Autodesk Fusion 360 part; units mm, degrees
note: some values were not read from the file. Set by a fixed rule: which sketch regions a step uses.
(part 2 of 2)
sketch "Lead ins" plane through (0, 0, 0) normal (0, 0, 1) x (1, 0, 0)
  line L0 (76.8702, 33.6176) -> (72.7083, 33.6176) construction
  line L1 (72.7083, 33.6176) -> (70, 33.6176)
  line L2 (-72.7083, 33.6176) -> (-76.8702, 33.6176) construction
  line L3 (-72.7083, 33.6176) -> (-70, 33.6176)
  line L4 (-70, 33.6176) -> (-70, 33.3926) construction
  line L5 (70, 33.6176) -> (70, 33.3926) construction
  line L6 (-72.7083, 8.1676) -> (-76.8702, 8.1676) construction
  arc A0 (-72.7083, 8.1676) -> (-68.9368, 10.4435) centre (-70, 7.9426) ccw construction
  arc A1 (-68.9368, 10.4435) -> (-72.7083, 8.1676) centre (-70, 7.9426) ccw construction
  arc A2 (-71.4041, 10.2693) -> (-72.7083, 8.1676) centre (-70, 7.9426) ccw
  line L7 (-72.7083, 8.1676) -> (-70, 8.1676)
  line L8 (-70, 7.9426) -> (-70, 8.1676) construction
  line L9 (76.8702, 8.1676) -> (72.7083, 8.1676) construction
  arc A3 (68.9368, 10.4435) -> (72.7083, 8.1676) centre (70, 7.9426) ccw construction
  line L10 (72.7083, 8.1676) -> (70, 8.1676)
  line L11 (70, 8.1676) -> (70, 7.9426) construction
  arc A4 (72.7083, 8.1676) -> (68.9368, 10.4435) centre (70, 7.9426) ccw construction
  arc A5 (72.7083, 8.1676) -> (71.4041, 10.2693) centre (70, 7.9426) ccw
  point P0 (-70, 33.3926)
  point P1 (70, 33.3926)
  point P2 (-70, 7.9426)
  point P3 (71.4041, 10.2693)
  constraint parallel L0 L1
  constraint coincident L2.start L3.start
  constraint parallel L2 L3
  constraint coincident P0 L4.end
  constraint perpendicular L3 L4
  constraint coincident P1 L5.end
  constraint perpendicular L1 L5
  constraint coincident L0.end L1.start
  constraint coincident L6.start A0.start
  constraint coincident A0.end A1.start
  constraint coincident P2 A0.centre
  constraint midpoint A1 A2.start
  constraint parallel L6 L7
  constraint perpendicular L7 L8
  constraint coincident L9.end A3.end
  constraint parallel L9 L10
  constraint coincident A3.centre L11.end
  constraint perpendicular L10 L11
  constraint coincident A3.start A4.end
  constraint midpoint A4 P3
  constraint coincident P3 A5.end
sketch "Cuts" plane through (0, 0, 0) normal (0, 0, 1) x (1, 0, 0)
  arc A0 (-60.4613, 48.9428) -> (-61.177, 48.6145) centre (-53.134, 32.0265) ccw
  line L0 (-61.177, 48.6145) -> (-61.2612, 48.783)
  arc A1 (-61.2612, 48.783) -> (-64.4705, 49.6307) centre (-63.2391, 47.794) ccw
  line L1 (-64.4705, 49.6307) -> (-66.6685, 48.1572)
  arc A2 (-66.6685, 48.1572) -> (-66.9278, 45.5047) centre (-65.7079, 46.7244) ccw
  line L2 (-66.9278, 45.5047) -> (-66.4745, 45.0513)
  line L3 (-66.4745, 45.0513) -> (-65.6771, 45.5859)
  line L4 (-65.6771, 45.5859) -> (-65.6567, 45.5555)
  arc A3 (-65.6567, 45.5555) -> (-70.2084, 38.9774) centre (-53.134, 32.0265) ccw
  arc A4 (-70.2084, 38.9774) -> (-68.9368, 35.8935) centre (-68.0067, 38.0811) ccw
  arc A5 (-72.7083, 33.6176) -> (-68.9368, 35.8935) centre (-70, 33.3926) ccw
  line L5 (-72.7083, 33.6176) -> (-76.8702, 33.6176)
  arc A6 (-76.8702, 33.6176) -> (-78.0824, 32.2161) centre (-76.8702, 32.3926) ccw
  arc A7 (-78.0824, 32.2161) -> (-70, 25.225) centre (-70, 33.3926) ccw
  line L6 (-70, 25.225) -> (-53.8183, 25.225)
  line L7 (-53.8183, 25.225) -> (-52.078, 25.5991)
  arc A8 (-52.078, 25.5991) -> (-51.2745, 26.1842) centre (-52.3354, 26.7967) ccw
  line L8 (-51.2745, 26.1842) -> (-50.3319, 27.817)
  arc A9 (-50.3319, 27.817) -> (-47.5143, 26.9115) centre (-46.5, 34.9039) ccw
  line L9 (-47.5143, 26.9115) -> (-45.4857, 26.9115)
  arc A10 (-45.4857, 26.9115) -> (-41.0636, 28.9581) centre (-46.5, 34.9039) ccw
  arc A11 (-41.0636, 28.9581) -> (-40.8293, 30.4746) centre (-41.8902, 29.8621) ccw
  line L10 (-40.8293, 30.4746) -> (-43.0033, 34.24)
  line L11 (-43.0033, 34.24) -> (-44.1175, 33.5967)
  arc A12 (-45.5402, 32.3615) -> (-44.1175, 33.5967) centre (-46.5, 34.9039) ccw
  line L12 (-45.5402, 32.3615) -> (-47.4598, 32.3615)
  arc A13 (-48.8317, 33.5081) -> (-47.4598, 32.3615) centre (-46.5, 34.9039) ccw
  arc A14 (-48.0318, 36.5907) -> (-48.8317, 33.5081) centre (-46.9147, 34.6557) ccw
  line L13 (-48.0318, 36.5907) -> (-43.7627, 39.0554)
  line L14 (-43.7627, 39.0554) -> (-39.2352, 31.2135)
  arc A15 (-39.2352, 31.2135) -> (-33.999, 28.6496) centre (-34.7102, 33.826) ccw
  arc A16 (-2.725, 30.9595) -> (-33.999, 28.6496) centre (0, -218.8006) ccw
  line L15 (-2.725, 30.9595) -> (-2.725, 31.7494)
  arc A17 (-1, 33.4744) -> (-2.725, 31.7494) centre (-1, 31.7494) ccw
  line L16 (-1, 33.4744) -> (1, 33.4744)
  arc A18 (2.725, 31.7494) -> (1, 33.4744) centre (1, 31.7494) ccw
  line L17 (2.725, 31.7494) -> (2.725, 30.9595)
  arc A19 (33.999, 28.6496) -> (2.725, 30.9595) centre (0, -218.8006) ccw
  arc A20 (33.999, 28.6496) -> (39.2352, 31.2135) centre (34.7102, 33.826) ccw
  line L18 (39.2352, 31.2135) -> (43.7627, 39.0554)
  line L19 (43.7627, 39.0554) -> (48.0318, 36.5907)
  arc A21 (48.8317, 33.5081) -> (48.0318, 36.5907) centre (46.9147, 34.6557) ccw
  arc A22 (47.4598, 32.3615) -> (48.8317, 33.5081) centre (46.5, 34.9039) ccw
  line L20 (47.4598, 32.3615) -> (45.5402, 32.3615)
  arc A23 (44.1175, 33.5967) -> (45.5402, 32.3615) centre (46.5, 34.9039) ccw
  line L21 (44.1175, 33.5967) -> (43.0033, 34.24)
  line L22 (43.0033, 34.24) -> (40.8293, 30.4746)
  arc A24 (40.8293, 30.4746) -> (41.0636, 28.9581) centre (41.8902, 29.8621) ccw
  arc A25 (41.0636, 28.9581) -> (45.4857, 26.9115) centre (46.5, 34.9039) ccw
  line L23 (45.4857, 26.9115) -> (47.5143, 26.9115)
  arc A26 (47.5143, 26.9115) -> (50.3319, 27.817) centre (46.5, 34.9039) ccw
  line L24 (50.3319, 27.817) -> (51.2745, 26.1842)
  arc A27 (51.2745, 26.1842) -> (52.078, 25.5991) centre (52.3354, 26.7967) ccw
  line L25 (52.078, 25.5991) -> (53.8183, 25.225)
  line L26 (53.8183, 25.225) -> (70, 25.225)
  arc A28 (70, 25.225) -> (78.0824, 32.2161) centre (70, 33.3926) ccw
  arc A29 (78.0824, 32.2161) -> (76.8702, 33.6176) centre (76.8702, 32.3926) ccw
  line L27 (76.8702, 33.6176) -> (72.7083, 33.6176)
  arc A30 (68.9368, 35.8935) -> (72.7083, 33.6176) centre (70, 33.3926) ccw
  arc A31 (68.9368, 35.8935) -> (70.2084, 38.9774) centre (68.0067, 38.0811) ccw
  arc A32 (70.2084, 38.9774) -> (65.6567, 45.5555) centre (53.134, 32.0265) ccw
  line L28 (65.6567, 45.5555) -> (65.6771, 45.5859)
  line L29 (65.6771, 45.5859) -> (66.4745, 45.0513)
  line L30 (66.4745, 45.0513) -> (66.9278, 45.5047)
  arc A33 (66.9278, 45.5047) -> (66.6685, 48.1572) centre (65.7079, 46.7244) ccw
  line L31 (66.6685, 48.1572) -> (64.4705, 49.6307)
  arc A34 (64.4705, 49.6307) -> (61.2612, 48.783) centre (63.2391, 47.794) ccw
  line L32 (61.2612, 48.783) -> (61.177, 48.6145)
  arc A35 (61.177, 48.6145) -> (60.4613, 48.9428) centre (53.134, 32.0265) ccw
  arc A36 (60.4613, 48.9428) -> (59.7108, 49.1956) centre (58.5833, 44.6071) ccw
  arc A37 (59.7108, 49.1956) -> (2.725, 56.4095) centre (0, -193.8006) ccw
  line L33 (2.725, 56.4095) -> (2.725, 57.1994)
  arc A38 (2.725, 57.1994) -> (1, 58.9244) centre (1, 57.1994) ccw
  line L34 (1, 58.9244) -> (-1, 58.9244)
  arc A39 (-1, 58.9244) -> (-2.725, 57.1994) centre (-1, 57.1994) ccw
  line L35 (-2.725, 57.1994) -> (-2.725, 56.4095)
  arc A40 (-59.7108, 49.1956) -> (-60.4613, 48.9428) centre (-58.5833, 44.6071) ccw
  arc A41 (-2.725, 56.4095) -> (-59.7108, 49.1956) centre (0, -193.8006) ccw
  arc A42 (-39.2352, 5.7635) -> (-33.999, 3.1996) centre (-34.7102, 8.376) ccw
  line L36 (-43.7627, 13.6054) -> (-39.2352, 5.7635)
  line L37 (-48.0318, 11.1407) -> (-43.7627, 13.6054)
  arc A43 (-48.0318, 11.1407) -> (-48.8317, 8.0581) centre (-46.9147, 9.2057) ccw
  arc A44 (-48.8317, 8.0581) -> (-47.4598, 6.9115) centre (-46.5, 9.4539) ccw
  line L38 (-45.5402, 6.9115) -> (-47.4598, 6.9115)
  arc A45 (-45.5402, 6.9115) -> (-44.1175, 8.1467) centre (-46.5, 9.4539) ccw
  line L39 (-43.0033, 8.79) -> (-44.1175, 8.1467)
  line L40 (-40.8293, 5.0246) -> (-43.0033, 8.79)
  arc A46 (-41.0636, 3.5081) -> (-40.8293, 5.0246) centre (-41.8902, 4.4121) ccw
  arc A47 (-45.4857, 1.4615) -> (-41.0636, 3.5081) centre (-46.5, 9.4539) ccw
  line L41 (-47.5143, 1.4615) -> (-45.4857, 1.4615)
  arc A48 (-50.3319, 2.367) -> (-47.5143, 1.4615) centre (-46.5, 9.4539) ccw
  line L42 (-51.2745, 0.7342) -> (-50.3319, 2.367)
  arc A49 (-52.078, 0.1491) -> (-51.2745, 0.7342) centre (-52.3354, 1.3467) ccw
  line L43 (-53.8183, -0.225) -> (-52.078, 0.1491)
  line L44 (-70, -0.225) -> (-53.8183, -0.225)
  arc A50 (-78.0824, 6.7661) -> (-70, -0.225) centre (-70, 7.9426) ccw
  arc A51 (-76.8702, 8.1676) -> (-78.0824, 6.7661) centre (-76.8702, 6.9426) ccw
  line L45 (-72.7083, 8.1676) -> (-76.8702, 8.1676)
  arc A52 (-72.7083, 8.1676) -> (-68.9368, 10.4435) centre (-70, 7.9426) ccw
  arc A53 (-70.2084, 13.5274) -> (-68.9368, 10.4435) centre (-68.0067, 12.6311) ccw
  arc A54 (-65.6567, 20.1055) -> (-70.2084, 13.5274) centre (-53.134, 6.5765) ccw
  line L46 (-65.6771, 20.1359) -> (-65.6567, 20.1055)
  line L47 (-66.4745, 19.6013) -> (-65.6771, 20.1359)
  line L48 (-66.9278, 20.0547) -> (-66.4745, 19.6013)
  arc A55 (-66.6685, 22.7072) -> (-66.9278, 20.0547) centre (-65.7079, 21.2744) ccw
  line L49 (-64.4705, 24.1807) -> (-66.6685, 22.7072)
  arc A56 (-61.2612, 23.333) -> (-64.4705, 24.1807) centre (-63.2391, 22.344) ccw
  line L50 (-61.177, 23.1645) -> (-61.2612, 23.333)
  arc A57 (-60.4613, 23.4928) -> (-61.177, 23.1645) centre (-53.134, 6.5765) ccw
  arc A58 (-59.7108, 23.7456) -> (-60.4613, 23.4928) centre (-58.5833, 19.1571) ccw
  arc A59 (60.4613, 23.4928) -> (59.7108, 23.7456) centre (58.5833, 19.1571) ccw
  arc A60 (61.177, 23.1645) -> (60.4613, 23.4928) centre (53.134, 6.5765) ccw
  line L51 (61.2612, 23.333) -> (61.177, 23.1645)
  arc A61 (64.4705, 24.1807) -> (61.2612, 23.333) centre (63.2391, 22.344) ccw
  line L52 (66.6685, 22.7072) -> (64.4705, 24.1807)
  arc A62 (66.9278, 20.0547) -> (66.6685, 22.7072) centre (65.7079, 21.2744) ccw
  line L53 (66.4745, 19.6013) -> (66.9278, 20.0547)
  line L54 (65.6771, 20.1359) -> (66.4745, 19.6013)
  line L55 (65.6567, 20.1055) -> (65.6771, 20.1359)
  arc A63 (70.2084, 13.5274) -> (65.6567, 20.1055) centre (53.134, 6.5765) ccw
  arc A64 (68.9368, 10.4435) -> (70.2084, 13.5274) centre (68.0067, 12.6311) ccw
  arc A65 (68.9368, 10.4435) -> (72.7083, 8.1676) centre (70, 7.9426) ccw
  line L56 (76.8702, 8.1676) -> (72.7083, 8.1676)
  arc A66 (78.0824, 6.7661) -> (76.8702, 8.1676) centre (76.8702, 6.9426) ccw
  arc A67 (70, -0.225) -> (78.0824, 6.7661) centre (70, 7.9426) ccw
  line L57 (53.8183, -0.225) -> (70, -0.225)
  line L58 (52.078, 0.1491) -> (53.8183, -0.225)
  arc A68 (51.2745, 0.7342) -> (52.078, 0.1491) centre (52.3354, 1.3467) ccw
  line L59 (50.3319, 2.367) -> (51.2745, 0.7342)
  arc A69 (47.5143, 1.4615) -> (50.3319, 2.367) centre (46.5, 9.4539) ccw
  line L60 (45.4857, 1.4615) -> (47.5143, 1.4615)
  arc A70 (41.0636, 3.5081) -> (45.4857, 1.4615) centre (46.5, 9.4539) ccw
  arc A71 (40.8293, 5.0246) -> (41.0636, 3.5081) centre (41.8902, 4.4121) ccw
  line L61 (43.0033, 8.79) -> (40.8293, 5.0246)
  line L62 (44.1175, 8.1467) -> (43.0033, 8.79)
  arc A72 (44.1175, 8.1467) -> (45.5402, 6.9115) centre (46.5, 9.4539) ccw
  line L63 (47.4598, 6.9115) -> (45.5402, 6.9115)
  arc A73 (47.4598, 6.9115) -> (48.8317, 8.0581) centre (46.5, 9.4539) ccw
  arc A74 (48.8317, 8.0581) -> (48.0318, 11.1407) centre (46.9147, 9.2057) ccw
  line L64 (43.7627, 13.6054) -> (48.0318, 11.1407)
  line L65 (39.2352, 5.7635) -> (43.7627, 13.6054)
  arc A75 (33.999, 3.1996) -> (39.2352, 5.7635) centre (34.7102, 8.376) ccw
  arc A76 (33.999, 3.1996) -> (2.725, 5.5095) centre (0, -244.2506) ccw
  line L66 (2.725, 6.2994) -> (2.725, 5.5095)
  arc A77 (2.725, 6.2994) -> (1, 8.0244) centre (1, 6.2994) ccw
  line L67 (-1, 8.0244) -> (1, 8.0244)
  arc A78 (-1, 8.0244) -> (-2.725, 6.2994) centre (-1, 6.2994) ccw
  line L68 (-2.725, 5.5095) -> (-2.725, 6.2994)
  arc A79 (-2.725, 5.5095) -> (-33.999, 3.1996) centre (0, -244.2506) ccw
  arc A80 (-2.725, 30.9595) -> (-59.7108, 23.7456) centre (0, -219.2506) ccw construction
  arc A81 (59.7108, 23.7456) -> (2.725, 30.9595) centre (0, -219.2506) ccw construction
  arc A82 (-34.3171, 28.61) -> (-59.7108, 23.7456) centre (0, -219.2506) ccw
  arc A83 (59.7108, 23.7456) -> (34.3171, 28.61) centre (0, -219.2506) ccw
  line L69 (72.7083, 8.1676) -> (70, 8.1676)
  arc A84 (72.7083, 8.1676) -> (71.4041, 10.2693) centre (70, 7.9426) ccw
  line L70 (72.7083, 33.6176) -> (70, 33.6176)
  point P0 (-34.2057, 28.6254)
  point P1 (-34.3171, 28.61)
  point P2 (34.2057, 28.6254)
  point P3 (34.3171, 28.61)
  dimension "d667" = 0.1125
  dimension "d668" = 0.1125
  constraint coincident A80 P0
  constraint coincident A15 P0
  constraint coincident A80 P1
  constraint coincident A58.start A80.end
  constraint coincident P1 A82.start
  constraint concentric A80 A82
  constraint coincident A20 P2
  constraint coincident A81 P2
  constraint coincident A81 P3
  constraint coincident P3 A83.end
  constraint coincident A59.end A81.start
  constraint concentric A81 A83
  measures "d667" distance of P0 P1
  measures "d668" distance of P2 P3
sketch "Sketch58" plane through (0, 0, 3) normal (0, 0, 1) x (-1, 0, 0)
sketch "Sketch59" plane through (0, 0, 3) normal (0, 0, 1) x (-1, 0, 0)
  line L0 (-2.95, -6.2994) -> (-2.95, -5.732)
  arc A0 (-34.0296, -3.4225) -> (-2.95, -5.732) centre (0, 244.2506) ccw
  arc A1 (-34.0296, -3.4225) -> (-39.0403, -5.876) centre (-34.7102, -8.376) ccw
  line L1 (-39.0403, -5.876) -> (-43.6804, -13.9128)
  line L2 (-43.6804, -13.9128) -> (-48.1443, -11.3355)
  arc A2 (-49.0248, -7.9426) -> (-48.1443, -11.3355) centre (-46.9147, -9.2057) ccw
  arc A3 (-47.5, -6.6865) -> (-49.0248, -7.9426) centre (-46.5, -9.4539) ccw
  line L3 (-47.5, -6.6865) -> (-45.5, -6.6865)
  arc A4 (-43.9516, -7.9827) -> (-45.5, -6.6865) centre (-46.5, -9.4539) ccw
  line L4 (-43.9516, -7.9827) -> (-43.0856, -8.4827)
  line L5 (-43.0856, -8.4827) -> (-41.0242, -4.9121)
  arc A5 (-41.0242, -4.9121) -> (-41.2154, -3.6741) centre (-41.8902, -4.4121) ccw
  arc A6 (-41.2154, -3.6741) -> (-45.5, -1.6865) centre (-46.5, -9.4539) ccw
  line L6 (-45.5, -1.6865) -> (-47.5, -1.6865)
  arc A7 (-47.5, -1.6865) -> (-50.4158, -2.6716) centre (-46.5, -9.4539) ccw
  line L7 (-50.4158, -2.6716) -> (-51.4694, -0.8467)
  arc A8 (-51.4694, -0.8467) -> (-52.1253, -0.3691) centre (-52.3354, -1.3467) ccw
  line L8 (-52.1253, -0.3691) -> (-53.8422, 0)
  line L9 (-53.8422, 0) -> (-70, 0)
  arc A9 (-70, 0) -> (-77.8598, -6.7985) centre (-70, -7.9426) ccw
  arc A10 (-77.8598, -6.7985) -> (-76.8702, -7.9426) centre (-76.8702, -6.9426) ccw
  line L10 (-76.8702, -7.9426) -> (-72.9426, -7.9426)
  arc A11 (-68.8487, -10.6506) -> (-72.9426, -7.9426) centre (-70, -7.9426) ccw
  arc A12 (-68.8487, -10.6506) -> (-70, -13.4426) centre (-68.0067, -12.6311) ccw
  arc A13 (-70, -13.4426) -> (-65.3622, -20.0701) centre (-53.134, -6.5765) ccw
  line L11 (-65.3622, -20.0701) -> (-65.6155, -20.4481)
  line L12 (-65.6155, -20.4481) -> (-66.4461, -19.8912)
  line L13 (-66.4461, -19.8912) -> (-66.7687, -20.2138)
  arc A14 (-66.7687, -20.2138) -> (-66.5432, -22.5203) centre (-65.7079, -21.2744) ccw
  line L14 (-66.5432, -22.5203) -> (-64.3452, -23.9939)
  arc A15 (-64.3452, -23.9939) -> (-61.4625, -23.2324) centre (-63.2391, -22.344) ccw
  line L15 (-61.4625, -23.2324) -> (-61.2782, -22.8639)
  arc A16 (-61.2782, -22.8639) -> (-60.3719, -23.2864) centre (-53.134, -6.5765) ccw
  arc A17 (-60.3719, -23.2864) -> (-59.6571, -23.5271) centre (-58.5833, -19.1571) ccw
  arc A18 (-59.6571, -23.5271) -> (-2.5, -30.7369) centre (0, 219.2506) ccw
  line L16 (-2.5, -30.7369) -> (-2.5, -31.7494)
  arc A19 (-2.5, -31.7494) -> (-1, -33.2494) centre (-1, -31.7494) ccw
  line L17 (-1, -33.2494) -> (1, -33.2494)
  arc A20 (1, -33.2494) -> (2.5, -31.7494) centre (1, -31.7494) ccw
  line L18 (2.5, -31.7494) -> (2.5, -30.7369)
  arc A21 (2.5, -30.7369) -> (59.6571, -23.5271) centre (0, 219.2506) ccw
  arc A22 (59.6571, -23.5271) -> (60.3719, -23.2864) centre (58.5833, -19.1571) ccw
  arc A23 (60.3719, -23.2864) -> (61.2782, -22.8639) centre (53.134, -6.5765) ccw
  line L19 (61.2782, -22.8639) -> (61.4625, -23.2324)
  arc A24 (61.4625, -23.2324) -> (64.3452, -23.9939) centre (63.2391, -22.344) ccw
  line L20 (64.3452, -23.9939) -> (66.5432, -22.5203)
  arc A25 (66.5432, -22.5203) -> (66.7687, -20.2138) centre (65.7079, -21.2744) ccw
  line L21 (66.7687, -20.2138) -> (66.4461, -19.8912)
  line L22 (66.4461, -19.8912) -> (65.6155, -20.4481)
  line L23 (65.6155, -20.4481) -> (65.3622, -20.0701)
  arc A26 (65.3622, -20.0701) -> (70, -13.4426) centre (53.134, -6.5765) ccw
  arc A27 (70, -13.4426) -> (68.8487, -10.6506) centre (68.0067, -12.6311) ccw
  arc A28 (72.9426, -7.9426) -> (68.8487, -10.6506) centre (70, -7.9426) ccw
  line L24 (72.9426, -7.9426) -> (76.8702, -7.9426)
  arc A29 (76.8702, -7.9426) -> (77.8598, -6.7985) centre (76.8702, -6.9426) ccw
  arc A30 (77.8598, -6.7985) -> (70, 0) centre (70, -7.9426) ccw
  line L25 (70, 0) -> (53.8422, 0)
  line L26 (53.8422, 0) -> (52.1253, -0.3691)
  arc A31 (52.1253, -0.3691) -> (51.4694, -0.8467) centre (52.3354, -1.3467) ccw
  line L27 (51.4694, -0.8467) -> (50.4158, -2.6716)
  arc A32 (50.4158, -2.6716) -> (47.5, -1.6865) centre (46.5, -9.4539) ccw
  line L28 (47.5, -1.6865) -> (45.5, -1.6865)
  arc A33 (45.5, -1.6865) -> (41.2154, -3.6741) centre (46.5, -9.4539) ccw
  arc A34 (41.2154, -3.6741) -> (41.0242, -4.9121) centre (41.8902, -4.4121) ccw
  line L29 (41.0242, -4.9121) -> (43.0856, -8.4827)
  line L30 (43.0856, -8.4827) -> (43.9516, -7.9827)
  arc A35 (45.5, -6.6865) -> (43.9516, -7.9827) centre (46.5, -9.4539) ccw
  line L31 (45.5, -6.6865) -> (47.5, -6.6865)
  arc A36 (49.0248, -7.9426) -> (47.5, -6.6865) centre (46.5, -9.4539) ccw
  arc A37 (48.1443, -11.3355) -> (49.0248, -7.9426) centre (46.9147, -9.2057) ccw
  line L32 (48.1443, -11.3355) -> (43.6804, -13.9128)
  line L33 (43.6804, -13.9128) -> (39.0403, -5.876)
  arc A38 (39.0403, -5.876) -> (34.0296, -3.4225) centre (34.7102, -8.376) ccw
  arc A39 (2.95, -5.732) -> (34.0296, -3.4225) centre (0, 244.2506) ccw
  line L34 (2.95, -5.732) -> (2.95, -6.2994)
  arc A40 (1, -8.2494) -> (2.95, -6.2994) centre (1, -6.2994) ccw
  line L35 (1, -8.2494) -> (-1, -8.2494)
  arc A41 (-2.95, -6.2994) -> (-1, -8.2494) centre (-1, -6.2994) ccw
component "Component" placed x (1, 0, 0) y (0, 1, 0) z (0, 0, 1) at (0, 0, 0)
component "Component" placed x (1, 0, 0) y (0, 1, 0) z (0, 0, 1) at (0, 25.45, 0)
equation "spike_depth = 2,5 mm"
equation "spike_fillet = 1,5 mm"
equation "spike_width = 5 mm"
equation "shield_thickness = 0,2 mm"
equation "bitragion_breath = 160 mm"
equation "d196 = spike_width"
equation "d198 = spike_fillet"
equation "d199 = spike_fillet"
equation "d314 = spike_depth"
equation "d321 = spike_fillet"
equation "d323 = spike_depth"
equation "d327 = spike_fillet"
equation "kerf = 0,45 mm"
equation "d450 = connection_circle_diameter"
equation "d457 = connection_circle_diameter"
equation "d459 = connector_height * 1 mm + ( connection_circle_diameter / 2 )"
equation "d463 = ( 140 / 2 ) * 1 mm"
equation "min_circle_diameter = ( sqrt(connector_height ^ 2 + connector_width ^ 2) ) * 1 mm"
equation "connector_width = 2"
equation "connector_height = 5"
equation "connection_circle_diameter = min_circle_diameter + 0,5 mm"
equation "d487 = connector_width * 1,1 mm"
equation "d522 = spike_depth"
equation "d527 = kerf"
equation "shield_slot_depth = 0,455 mm"
equation "d553 = shield_slot_depth"
equation "d554 = shield_slot_depth"
equation "d571 = connector_height * 1 mm"
equation "d575 = connection_circle_diameter / 2"
equation "d577 = connector_width * 1 mm / 2"
equation "d578 = connector_width * 0,5 mm"
equation "d579 = connection_circle_diameter / 2"
equation "d617 = connection_circle_diameter / 2"
equation "d618 = connector_width * 1 mm"
equation "d624 = connector_height * 1 mm"
equation "d634 = connector_width * 1,1 mm"
equation "d658 = kerf / 4"
equation "d664 = kerf / 4"
equation "d665 = kerf / 2"
equation "d666 = kerf / 2"
equation "d667 = kerf / 4"
equation "d668 = kerf / 4"
